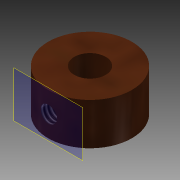
# Autodesk Inventor part: 13_1087_022
Saved by Autodesk Inventor 2014 (Build 180170000, 170)
## iProperties
Created: 2013-09-10
Part Number: 13_1087_022
Material: Allgemein
Document SubType Name: Modeling
Designer: vogel
Density: 1 g/cm^3
Appearance: Walnuss - natur - poliert
Author: vogel
Autodesk Inventor part; units mm, degrees
note: some values were not read from the file. Chosen so that the rebuilt part matches the saved one: direction of "Bohrung1".
ref_plane "YZ Plane" through (0, 0, 0) normal (1, 0, 0) x (0, 1, 0)
ref_plane "XY Plane" through (0, 0, 0) normal (0, 0, 1) x (1, 0, 0)
sketch "Skizze1" plane through (0, 0, 0) normal (0, 0, 1) x (1, 0, 0)
  line L0 (-5.6, 0) -> (5.6, 0) projected
  line L1 (0, -5.6) -> (0, 5.6) projected
  circle A0 centre (0, 0) radius 1.5
  circle A1 centre (0, 0) radius 4
  dimension "d0" = 3
  dimension "d1" = 8
  constraints: 2 centre point, 2 coincident
  measures "d0" diameter of A0
  measures "d1" diameter of A1
extrude "Extrusion1" add sketch "Skizze1" along normal blind 4 contours A0 L1 A1 L0 | L0 A1 L1 A0 | A0 L0 A1 L1 | L1 A1 L0 A0
ref_plane "Arbeitsebene1" through (0, -4, 0) normal (0, 1, 0) x (-1, 0, 0)
sketch "Skizze2" plane through (0, -4, 0) normal (0, 1, 0) x (-1, 0, 0)
  line L0 (0, -0.8) -> (0, 4.8) projected
  line L1 (5.6, 0) -> (-5.6, 0) projected
  point P0 (0, 0)
  point P1 (0, 2)
  dimension "d4" = 2
  constraints: 1 midpoint
  measures "d4" distance from line of L1 point (0, 2)
hole "Bohrung1" at (0, -4, 2) direction (0, 1, 0) diameter 1.567 end up to surface thread size "M2x0.4" class "6H" standard "ISO Metric profile"
